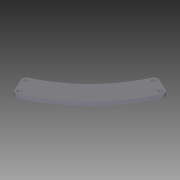
# Autodesk Inventor part: motorplate
Saved by Autodesk Inventor 2015 (Build 190159000, 159)
## iProperties
Created: 2015-02-25
Part Number: motorplate
Material: Generic
Document SubType Name: Modeling
Designer: janov_000
Density: 1 g/cm^3
Appearance: Aluminum - Flat
Author: janov_000
Autodesk Inventor part; units mm, degrees
ref_plane "YZ Plane" through (0, 0, 0) normal (1, 0, 0) x (0, 1, 0)
ref_plane "XZ Plane" through (0, 0, 0) normal (0, 1, 0) x (-1, 0, 0)
ref_plane "XY Plane" through (0, 0, 0) normal (0, 0, 1) x (1, 0, 0)
sketch "Sketch1" plane through (0, 0, 0) normal (0, 0, 1) x (1, 0, 0)
  circle A0 centre (-3.6979, 7.9302) radius 2.5 projected
  circle A1 centre (3.6979, -7.9302) radius 2.5 projected
  line L0 (-8.2294, 5.8171) -> (-0.8336, -10.0433) projected
  arc A2 (-0.8336, -10.0433) -> (8.2294, -5.8171) centre (3.6979, -7.9302) ccw projected
  line L1 (8.2294, -5.8171) -> (0.8336, 10.0433) projected
  arc A3 (0.8336, 10.0433) -> (-8.2294, 5.8171) centre (-3.6979, 7.9302) ccw projected
  circle A4 centre (78.5293, 90.1574) radius 2.5 projected
  circle A5 centre (94.3897, 82.7616) radius 2.5 projected
  line L2 (76.4162, 85.6259) -> (92.2766, 78.2301) projected
  arc A6 (92.2766, 78.2301) -> (96.5028, 87.2931) centre (94.3897, 82.7616) ccw projected
  line L3 (96.5028, 87.2931) -> (80.6424, 94.689) projected
  arc A7 (80.6424, 94.689) -> (76.4162, 85.6259) centre (78.5293, 90.1574) ccw projected
  circle A8 centre (-75.543, 162.0025) radius 75 projected
  circle A9 centre (-75.543, 162.0025) radius 170 construction
  arc A10 (-5.811, 12.4617) -> (73.9978, 92.2705) centre (-75.543, 162.0025) ccw
  arc A11 (5.811, -12.4617) -> (98.9212, 80.6485) centre (-75.543, 162.0025) ccw
  line L4 (-8.2294, 5.8171) -> (-0.8336, -10.0433)
  line L5 (80.6424, 94.689) -> (96.5028, 87.2931)
  arc A12 (80.6424, 94.689) -> (73.9978, 92.2705) centre (78.5293, 90.1574) ccw
  arc A13 (98.9212, 80.6485) -> (96.5028, 87.2931) centre (94.3897, 82.7616) ccw
  arc A14 (-5.811, 12.4617) -> (-8.2294, 5.8171) centre (-3.6979, 7.9302) ccw
  arc A15 (-0.8336, -10.0433) -> (5.811, -12.4617) centre (3.6979, -7.9302) ccw
  point P0 (0, 0)
  point P1 (-10.3746, 10.4173)
  point P2 (1.252, -14.516)
  point P3 (76.0422, 96.8341)
  point P4 (100.9755, 85.2075)
  dimension "d1" = 330
  dimension "d2" = 385
  dimension "d3" = 5
  dimension "d4" = 5
  dimension "d5" = 5
  dimension "d6" = 5
  dimension "d7" = 5
  constraints: 16 point on circle, 8 tangent, 7 coincident, 6 centre point, 4 end point, 4 point on line, 3 equal radius, 3 other
  measures "d1" diameter of A10
  measures "d2" diameter of A11
  measures "d3" distance from line of L4 A1.centre
  measures "d4" distance from line of L4 A0.centre
  measures "d5" distance from line of L5 point (78.529, 90.157)
  measures "d6" distance from line of A5.centre L5
  measures "d7" radius of A12
extrude "Extrusion1" add sketch "Sketch1" along normal blind 5 contours A0 | A1 | A3 L1 A2 L0 | A10 A7 L2 A6 A11 A2 L1 A3 | A7 L3 A6 L2 | A4 | A5
sketch "Sketch2" plane through (0, 0, 5) normal (0, 0, 1) x (1, 0, 0)
  circle A0 centre (-3.6979, 7.9302) radius 2.5 projected
  circle A1 centre (3.6979, -7.9302) radius 2.5 projected
  circle A2 centre (78.5293, 90.1574) radius 2.5 projected
  circle A3 centre (94.3897, 82.7616) radius 2.5 projected
  arc A4 (80.6424, 94.689) -> (73.9978, 92.2705) centre (78.5293, 90.1574) ccw projected
  arc A5 (-5.811, 12.4617) -> (-8.2294, 5.8171) centre (-3.6979, 7.9302) ccw projected
  point P0 (0, 0)
  constraints: 4 coincident
hole "Hole1" at (78.5293, 90.1574, 5) at (94.3897, 82.7616, 5) at (-3.6979, 7.9302, 5) at (3.6979, -7.9302, 5) direction (0, 0, -1) diameter 5 end through all
sketch "Sketch4" plane through (0, 0, 5) normal (0, 0, 1) x (1, 0, 0)
  circle A0 centre (23.1121, 21.1084) radius 10
  circle A1 centre (-3.6979, 7.9302) radius 2.5 projected
  circle A2 centre (78.5293, 90.1574) radius 2.5 projected
  circle A3 centre (94.3897, 82.7616) radius 2.5 projected
  circle A4 centre (3.6979, -7.9302) radius 2.5 projected
  arc A5 (80.6424, 94.689) -> (73.9978, 92.2705) centre (78.5293, 90.1574) ccw projected
  arc A6 (-5.811, 12.4617) -> (73.9978, 92.2705) centre (-75.543, 162.0025) ccw projected
  arc A7 (-5.811, 12.4617) -> (-8.2294, 5.8171) centre (-3.6979, 7.9302) ccw projected
  line L0 (-8.2294, 5.8171) -> (-0.8336, -10.0433) projected
  arc A8 (-0.8336, -10.0433) -> (5.811, -12.4617) centre (3.6979, -7.9302) ccw projected
  arc A9 (5.811, -12.4617) -> (98.9212, 80.6485) centre (-75.543, 162.0025) ccw projected
  arc A10 (98.9212, 80.6485) -> (96.5028, 87.2931) centre (94.3897, 82.7616) ccw projected
  line L1 (96.5028, 87.2931) -> (80.6424, 94.689) projected
  circle A11 centre (-75.543, 162.0025) radius 160 projected
  line L2 (-75.543, 162.0025) -> (23.1121, 21.1084) construction
  line L3 (-75.543, 162.0025) -> (-3.6979, 7.9302) construction
  line L4 (78.5293, 90.1574) -> (-75.543, 162.0025) construction
  arc A12 (-5.811, 12.4617) -> (73.9978, 92.2705) centre (-75.543, 162.0025) ccw projected
  line L5 (-75.543, 162.0025) -> (67.0687, 62.1447) construction
  point P0 (0, 0)
  dimension "d18" = 20
  dimension "d19" = 172
  dimension "d27" = 10
  dimension "d28" = 10
  constraints: 8 end point, 2 coincident, 1 centre point
  measures "d18" diameter of A0
  measures "d19" distance of L2.start L2.end
  measures "d27" angle of L2 L3
  measures "d28" angle of L4 L5
hole "Hole2" at (23.1121, 21.1084, 5) at (67.0687, 62.1447, 5) direction (0, 0, -1) diameter 10 end through all
sketch "Sketch6" plane through (0, 0, 5) normal (0, 0, 1) x (1, 0, 0)
  circle A0 centre (23.1121, 21.1084) radius 5 projected
  circle A1 centre (67.0687, 62.1447) radius 5 projected
  circle A2 centre (-3.6979, 7.9302) radius 2.5 projected
  circle A3 centre (78.5293, 90.1574) radius 2.5 projected
  circle A4 centre (94.3897, 82.7616) radius 2.5 projected
  circle A5 centre (3.6979, -7.9302) radius 2.5 projected
  arc A6 (80.6424, 94.689) -> (73.9978, 92.2705) centre (78.5293, 90.1574) ccw projected
  arc A7 (-5.811, 12.4617) -> (73.9978, 92.2705) centre (-75.543, 162.0025) ccw projected
  arc A8 (-5.811, 12.4617) -> (-8.2294, 5.8171) centre (-3.6979, 7.9302) ccw projected
  line L0 (-8.2294, 5.8171) -> (-0.8336, -10.0433) projected
  arc A9 (-0.8336, -10.0433) -> (5.811, -12.4617) centre (3.6979, -7.9302) ccw projected
  arc A10 (5.811, -12.4617) -> (98.9212, 80.6485) centre (-75.543, 162.0025) ccw projected
  arc A11 (98.9212, 80.6485) -> (96.5028, 87.2931) centre (94.3897, 82.7616) ccw projected
  line L1 (96.5028, 87.2931) -> (80.6424, 94.689) projected
  line L2 (23.1121, 21.1084) -> (7.9578, 10.4972) construction
  line L3 (23.1121, 21.1084) -> (38.2664, 31.7195) construction
  line L4 (23.1121, 21.1084) -> (19.0971, 26.8424)
  arc A12 (-5.811, 12.4617) -> (73.9978, 92.2705) centre (-75.543, 162.0025) ccw projected
  line L5 (67.0687, 62.1447) -> (56.4575, 46.9904)
  line L6 (67.0687, 62.1447) -> (77.6799, 77.299)
  line L7 (67.0687, 62.1447) -> (59.6171, 67.3624)
  point P0 (0, 0)
  dimension "d29" = 18.5
  dimension "d30" = 18.5
  dimension "d38" = 18.5
  dimension "d39" = 18.5
  constraints: 12 end point, 4 coincident, 4 point on circle, 2 collinear, 2 line through centre, 2 perpendicular
  measures "d29" distance of L2.start L2.end
  measures "d30" distance of L2.start L3.end
  measures "d38" distance of L5.start L5.end
  measures "d39" distance of L5.start L6.end
hole "Hole3" at (7.9578, 10.4972, 5) at (38.2664, 31.7195, 5) at (56.4575, 46.9904, 5) at (77.6799, 77.299, 5) direction (0, 0, -1) diameter 4.134 end through all thread size "M5x0.8" class "6H" standard "ANSI Metric M Profile"
body "Solid1"
